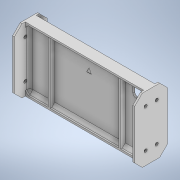
# Autodesk Inventor part: screen cover backplate
Saved by Autodesk Inventor 2021 (Build 250183000, 183)
## iProperties
Created: 2022-01-29
Part Number: screen cover backplate
Material: Generic
Document SubType Name: Modeling
Designer: Toby
Density: 1 g/cm^3
Appearance: Default
Author: Toby
Autodesk Inventor part; units mm, degrees
ref_plane "YZ Plane" through (0, 0, 0) normal (1, 0, 0) x (0, 1, 0)
ref_plane "XZ Plane" through (0, 0, 0) normal (0, 1, 0) x (-1, 0, 0)
ref_plane "XY Plane" through (0, 0, 0) normal (0, 0, 1) x (1, 0, 0)
sketch "Sketch1" plane through (0, 0, 0) normal (0, 0, 1) x (1, 0, 0)
  line L0 (-49.4736, 23.6675) -> (30.5264, 23.6675)
  line L1 (30.5264, 23.6675) -> (30.5264, -18.3325)
  line L2 (30.5264, -18.3325) -> (-49.4736, -18.3325)
  line L3 (-49.4736, -18.3325) -> (-49.4736, 23.6675)
  line L4 (-47.9736, 22.4675) -> (29.0264, 22.4675)
  line L5 (29.0264, 22.4675) -> (29.0264, -17.1325)
  line L6 (29.0264, -17.1325) -> (-47.9736, -17.1325)
  line L7 (-47.9736, -17.1325) -> (-47.9736, 22.4675)
  point P0 (0, 0)
  dimension "d0" = 80
  dimension "d1" = 42
  dimension "d2" = 1.5
  dimension "d3" = 1.5
  dimension "d4" = 1.2
  dimension "d5" = 1.2
  constraints: 16 end point, 4 parallel, 2 horizontal, 2 perpendicular
  measures "d0" distance of L0.start L0.end
  measures "d1" distance of L2.end L0.start
  measures "d2" distance between parallel lines of L7 L3
  measures "d3" distance between parallel lines of L1 L5
  measures "d4" distance between parallel lines of L0 L4
  measures "d5" distance between parallel lines of L2 L6
extrude "Extrusion1" add sketch "Sketch1" along normal blind 10
sketch "Sketch2" plane through (0, 0, 10) normal (0, 0, 1) x (1, 0, 0)
  line L0 (-47.9736, -18.3325) -> (29.0264, -18.3325)
  line L1 (29.0264, -18.3325) -> (29.0264, 23.6675)
  line L2 (29.0264, 23.6675) -> (-47.9736, 23.6675)
  line L3 (-47.9736, 23.6675) -> (-47.9736, -18.3325)
  line L4 (-47.9736, -17.1325) -> (-47.9736, 22.4675) projected
  line L5 (29.0264, 22.4675) -> (29.0264, -17.1325) projected
  line L6 (30.5264, 23.6675) -> (-49.4736, 23.6675) projected
  line L7 (-49.4736, -18.3325) -> (30.5264, -18.3325) projected
  point P0 (0, 0)
  constraints: 8 end point, 4 collinear, 2 parallel, 1 horizontal, 1 perpendicular
extrude "Extrusion2" cut sketch "Sketch2" against normal blind 10
sketch "Sketch3" plane through (0, 0, 10) normal (0, 0, 1) x (1, 0, 0)
  line L0 (-60.7413, 24.2408) -> (-49.3736, 24.2408)
  line L1 (-49.3736, 24.2408) -> (-49.3736, -19.8756)
  line L2 (-49.3736, -19.8756) -> (-60.7413, -19.8756)
  line L3 (-60.7413, -19.8756) -> (-60.7413, 24.2408)
  line L4 (46.8098, -23.8693) -> (30.4264, -23.8693)
  line L5 (30.4264, -23.8693) -> (30.4264, 25.2624)
  line L6 (30.4264, 25.2624) -> (46.8098, 25.2624)
  line L7 (46.8098, 25.2624) -> (46.8098, -23.8693)
  line L8 (-49.4736, 23.6675) -> (-49.4736, -18.3325) projected
  line L9 (30.5264, -18.3325) -> (30.5264, 23.6675) projected
  point P0 (0, 0)
  dimension "d10" = 0.1
  dimension "d11" = 0.1
  constraints: 16 end point, 4 parallel, 2 horizontal, 2 perpendicular
  measures "d10" distance between parallel lines of L1 L8
  measures "d11" distance between parallel lines of L9 L5
extrude "Extrusion3" cut sketch "Sketch3" against normal blind 10
sketch "Sketch4" plane through (30.4264, -18.3325, 10) normal (1, 0, 0) x (0, 0, -1)
  line L0 (10, 42) -> (10, 0) projected
  line L1 (0, 42) -> (10, 42) projected
  line L2 (10, 0) -> (0, 0) projected
  point P0 (10, 18.3325)
  point P1 (7, 33.5)
  point P2 (7, 8.5)
  dimension "d14" = 3
  dimension "d15" = 3
  dimension "d16" = 8.5
  dimension "d17" = 8.5
  measures "d14" distance from line of L0 point (7, 33.5)
  measures "d15" distance from line of L0 point (7, 8.5)
  measures "d16" distance from line of L1 point (7, 33.5)
  measures "d17" distance from line of L2 point (7, 8.5)
hole "Hole1" at (30.4264, 15.1675, 3) at (30.4264, -9.8325, 3) direction (-1, 0, 0) diameter 2 depth 10 tip angle 179
sketch "Sketch5" plane through (-49.3736, -18.3325, 10) normal (-1, 0, 0) x (0, 0, 1)
  circle A0 centre (-7, 33.5) radius 1 projected
  circle A1 centre (-7, 8.5) radius 1 projected
  point P0 (-10, 18.3325)
  constraints: 2 coincident
hole "Hole2" at (-49.3736, 15.1675, 3) at (-49.3736, -9.8325, 3) direction (1, 0, 0) diameter 2 depth 10 tip angle 179
chamfer "Chamfer1" distance 5 angle 45 4 edges at (-48.6736, 23.6675, 10) (-48.6736, -18.3325, 10) (29.7264, -18.3325, 10) (29.7264, 23.6675, 10)
sketch "Sketch6" plane through (0, 0, 0) normal (0, 0, -1) x (-1, 0, 0)
  line L0 (-30.4264, 23.6675) -> (-30.4264, -18.3325) projected
  line L1 (49.3736, -18.3325) -> (47.9736, -18.3325) projected
  line L2 (-30.4264, 23.6675) -> (49.3736, 23.6675)
  line L3 (49.3736, 23.6675) -> (49.3736, -18.3325)
  line L4 (49.3736, -18.3325) -> (-30.4264, -18.3325)
  line L5 (-30.4264, -18.3325) -> (-30.4264, 23.6675)
  point P0 (0, 0)
  point P1 (-30.4264, -18.3325)
  constraints: 8 end point, 2 parallel, 1 horizontal, 1 perpendicular
extrude "Extrusion4" add sketch "Sketch6" along normal blind 1.2
sketch "Sketch7" plane through (0, 0, -1.2) normal (0, 0, -1) x (-1, 0, 0)
  line L0 (-29.0264, -18.3325) -> (-29.0264, 23.6675) projected
  line L1 (-29.0264, 23.6675) -> (-19.0264, 23.6675)
  line L2 (-19.0264, 23.6675) -> (-19.0264, 13.6675)
  line L3 (-19.0264, 13.6675) -> (-29.0264, 13.6675)
  line L4 (-29.0264, 13.6675) -> (-29.0264, 23.6675)
  point P0 (0, 0)
  dimension "d37" = 10
  dimension "d38" = 10
  constraints: 8 end point, 2 parallel, 1 horizontal, 1 perpendicular
  measures "d37" distance of L2.end L3.end
  measures "d38" distance of L1.end L2.end
extrude "Extrusion5" cut sketch "Sketch7" against normal blind 1.2
fillet "Fillet1" radius 2 2 edges at (19.0264, 13.6675, -0.6) (29.0264, 13.6675, -0.6)
sketch "Sketch9" plane through (0, 0, 0) normal (0, 0, 1) x (1, 0, 0)
  line L0 (42.1128, -25.2677) -> (-53.8311, -25.2677)
  line L1 (-53.8311, -25.2677) -> (-53.8311, -18.2325)
  line L2 (-53.8311, -18.2325) -> (42.1128, -18.2325)
  line L3 (42.1128, -18.2325) -> (42.1128, -25.2677)
  line L4 (-54.7833, 25.6339) -> (39.9156, 25.6339)
  line L5 (39.9156, 25.6339) -> (39.9156, 23.5675)
  line L6 (39.9156, 23.5675) -> (-54.7833, 23.5675)
  line L7 (-54.7833, 23.5675) -> (-54.7833, 25.6339)
  line L8 (29.0264, -18.3325) -> (-47.9736, -18.3325) projected
  line L9 (-47.9736, 23.6675) -> (19.0264, 23.6675) projected
  point P0 (0, 0)
  dimension "d56" = 0.1
  dimension "d57" = 0.1
  constraints: 16 end point, 4 parallel, 2 horizontal, 2 perpendicular
  measures "d56" distance between parallel lines of L2 L8
  measures "d57" distance between parallel lines of L9 L6
extrude "Extrusion7" cut sketch "Sketch9" along normal mid plane 50
fillet "Fillet2" radius 2 2 edges at (-47.9736, 2.6675, 0) (29.0264, -1.2825, 0)
sketch "Sketch10" plane through (0, 0, 0) normal (0, 0, 1) x (1, 0, 0)
  line L0 (-47.9736, 23.5675) -> (-47.9736, 15.1675) projected
  line L1 (19.0264, 23.5675) -> (19.0264, 15.6675) projected
  line L2 (-47.9736, 23.5675) -> (19.0264, 23.5675)
  line L3 (19.0264, 23.5675) -> (19.0264, 22.4717)
  line L4 (19.0264, 22.4717) -> (-47.9736, 22.4717)
  line L5 (-47.9736, 22.4717) -> (-47.9736, 23.5675)
  line L6 (29.0264, -18.2325) -> (29.0264, -9.8325) projected
  line L7 (-47.9736, -9.8325) -> (-47.9736, -18.2325) projected
  line L8 (29.0264, -18.2325) -> (-47.9736, -18.2325)
  line L9 (-47.9736, -18.2325) -> (-47.9736, -17.0297)
  line L10 (-47.9736, -17.0297) -> (29.0264, -17.0297)
  line L11 (29.0264, -17.0297) -> (29.0264, -18.2325)
  point P0 (0, 0)
  point P1 (29.0264, -17.0297)
  constraints: 16 end point, 4 parallel, 2 horizontal, 2 perpendicular, 2 point on line
extrude "Extrusion8" add sketch "Sketch10" along normal blind 3
sketch "Sketch13" plane through (0, 0, -1.2) normal (0, 0, -1) x (-1, 0, 0)
  line L0 (-31.9264, 25.0675) -> (50.8736, 25.0675)
  line L1 (50.8736, 25.0675) -> (50.8736, -19.7325)
  line L2 (50.8736, -19.7325) -> (-31.9264, -19.7325)
  line L3 (-31.9264, -19.7325) -> (-31.9264, 25.0675)
  line L4 (49.3736, 23.5675) -> (-19.0264, 23.5675) projected
  line L5 (-30.4264, -18.2325) -> (49.3736, -18.2325) projected
  line L6 (-30.4264, 23.5675) -> (-30.4264, -18.2325) projected
  line L7 (49.3736, -18.2325) -> (49.3736, 23.5675) projected
  line L8 (-30.4264, 23.5675) -> (49.3736, 23.5675)
  line L9 (49.3736, 23.5675) -> (49.3736, -18.2325)
  line L10 (49.3736, -18.2325) -> (-30.4264, -18.2325)
  line L11 (-30.4264, -18.2325) -> (-30.4264, 23.5675)
  point P0 (0, 0)
  dimension "d81" = 1.5
  dimension "d82" = 1.5
  dimension "d83" = 1.5
  dimension "d84" = 1.5
  constraints: 16 end point, 4 parallel, 2 horizontal, 2 perpendicular
  measures "d81" distance between parallel lines of L4 L0
  measures "d82" distance between parallel lines of L2 L5
  measures "d83" distance between parallel lines of L6 L3
  measures "d84" distance between parallel lines of L7 L1
extrude "Extrusion11" add sketch "Sketch13" against normal blind 1.2
fillet "Fillet3" radius 2 3 edges at (31.9264, 25.0675, -0.6) (-50.8736, 25.0675, -0.6) (31.9264, -19.7325, -0.6)
fillet "Fillet4" radius 2 1 edges at (-50.8736, -19.7325, -0.6)
sketch "Sketch14" plane through (0, 0, -1.2) normal (0, 0, -1) x (-1, 0, 0)
  line L0 (-30.4264, 23.5675) -> (-29.0264, 23.5675) projected
  line L1 (-30.4264, -18.2325) -> (-30.4264, 23.5675) projected
  line L2 (-29.0264, 23.5675) -> (-30.4264, 23.5675)
  line L3 (-30.4264, 23.5675) -> (-30.4264, -18.2325)
  line L4 (-30.4264, -18.2325) -> (-29.0264, -18.2325)
  line L5 (-29.0264, -18.2325) -> (-29.0264, 23.5675)
  line L6 (49.3736, -18.2325) -> (47.9736, -18.2325) projected
  line L7 (49.3736, 23.5675) -> (49.3736, -18.2325) projected
  line L8 (47.9736, -18.2325) -> (49.3736, -18.2325)
  line L9 (49.3736, -18.2325) -> (49.3736, 23.5675)
  line L10 (49.3736, 23.5675) -> (47.9736, 23.5675)
  line L11 (47.9736, 23.5675) -> (47.9736, -18.2325)
  line L12 (-31.9264, 23.0675) -> (-31.9264, -17.7325) projected
  line L13 (48.8736, 25.0675) -> (-29.9264, 25.0675) projected
  point P0 (0, 0)
  dimension "d89" = 1.5
  dimension "d90" = 1.5
  constraints: 16 end point, 4 parallel, 2 horizontal, 2 perpendicular
  measures "d89" distance between parallel lines of L12 L1
  measures "d90" distance from line of L13 L0.start
extrude "Extrusion12" add sketch "Sketch14" along normal blind 10
sketch "Sketch15" plane through (30.4264, -18.2325, -1.2) normal (1, 0, 0) x (0, 0, -1)
  line L0 (0, 41.8) -> (10, 41.8) projected
  line L1 (0, 0) -> (10, 0) projected
  line L2 (0, 41.3) -> (0, 0.5) projected
  point P0 (-1.2, 18.2325)
  point P1 (3, 33.3)
  point P2 (3, 8.5)
  point P3 (5, 41.8)
  point P4 (5, 0)
  dimension "d96" = 8.5
  dimension "d97" = 8.5
  dimension "d98" = 3
  dimension "d99" = 3
  measures "d96" distance from line of L0 point (3, 33.3)
  measures "d97" distance from line of L1 point (3, 8.5)
  measures "d98" distance from line of L2 point (3, 8.5)
  measures "d99" distance from line of L2 point (3, 33.3)
hole "Hole3" at (30.4264, 15.0675, -4.2) at (30.4264, -9.7325, -4.2) direction (-1, 0, 0) diameter 2 depth 10 tip angle 179
sketch "Sketch16" plane through (-49.3736, -18.2325, -1.2) normal (-1, 0, 0) x (0, 0, 1)
  circle A0 centre (-3, 33.3) radius 1 projected
  circle A1 centre (-3, 8.5) radius 1 projected
  point P0 (1.2, 18.2325)
  constraints: 2 coincident
hole "Hole4" at (-49.3736, 15.0675, -4.2) at (-49.3736, -9.7325, -4.2) direction (1, 0, 0) diameter 2 depth 10 tip angle 179
chamfer "Chamfer4" distance 5 angle 45 4 edges at (29.7264, 23.5675, -11.2) (-48.6736, 23.5675, -11.2) (29.7264, -18.2325, -11.2) (-48.6736, -18.2325, -11.2)
chamfer "Chamfer5" distance 2 angle 45 5 edges at (-9.4736, -17.0297, 0) (28.4408, -17.0297, 0.5856) (29.0264, -17.0297, 2.4998) (-47.3879, -17.0297, 0.5856) (-47.9736, -17.0297, 2.4998)
chamfer "Chamfer6" distance 2 angle 45 2 edges at (-13.4738, 22.4717, 0) (-47.3879, 22.4717, 0.5856)
sketch "Sketch17" plane through (0, 0, -1.2) normal (0, 0, -1) x (-1, 0, 0)
  line L0 (-19.0264, 23.5675) -> (47.9736, 23.5675) projected
  line L1 (47.9736, 23.5675) -> (-19.0264, 23.5675)
  line L2 (-19.0264, 23.5675) -> (-19.0264, 22.3675)
  line L3 (-19.0264, 22.3675) -> (47.9736, 22.3675)
  line L4 (47.9736, 22.3675) -> (47.9736, 23.5675)
  line L5 (-29.0264, -15.0297) -> (-29.0264, -18.2325) projected
  line L6 (-29.0264, -18.2325) -> (47.9736, -18.2325)
  line L7 (47.9736, -18.2325) -> (47.9736, -17.0325)
  line L8 (47.9736, -17.0325) -> (-29.0264, -17.0325)
  line L9 (-29.0264, -17.0325) -> (-29.0264, -18.2325)
  line L10 (-19.0264, 23.5675) -> (-19.0264, 15.6675) projected
  point P0 (0, 0)
  point P1 (-29.0264, -17.0325)
  dimension "d123" = 1.2
  dimension "d124" = 1.2
  constraints: 16 end point, 4 parallel, 2 horizontal, 2 perpendicular, 1 collinear, 1 point on line
  measures "d123" distance between parallel lines of L3 L0
  measures "d124" distance between parallel lines of L6 L8
extrude "Extrusion13" add sketch "Sketch17" along normal blind 3
chamfer "Chamfer7" distance 2 angle 45 1 edges at (-14.4736, 22.3675, -1.2)
chamfer "Chamfer8" distance 2 angle 45 1 edges at (-9.4736, -17.0325, -1.2)
sketch "Sketch19" plane through (0, 0, -1.2) normal (0, 0, -1) x (-1, 0, 0)
  line L0 (-30.4264, -18.2325) -> (-30.4264, 23.5675) projected
  line L1 (47.9736, -18.2325) -> (49.3736, -18.2325) projected
  line L2 (-30.4264, 23.5675) -> (49.3736, 23.5675)
  line L3 (49.3736, 23.5675) -> (49.3736, -18.2325)
  line L4 (49.3736, -18.2325) -> (-30.4264, -18.2325)
  line L5 (-30.4264, -18.2325) -> (-30.4264, 23.5675)
  line L6 (55.2974, -21.7914) -> (-35.5213, -21.7914)
  line L7 (-35.5213, -21.7914) -> (-35.5213, 27.2078)
  line L8 (-35.5213, 27.2078) -> (55.2974, 27.2078)
  line L9 (55.2974, 27.2078) -> (55.2974, -21.7914)
  point P0 (0, 0)
  constraints: 16 end point, 4 parallel, 2 horizontal, 2 perpendicular
extrude "Extrusion14" cut sketch "Sketch19" against normal blind 3
sketch "Sketch20" plane through (0, 0, -1.2) normal (0, 0, -1) x (-1, 0, 0)
  line L0 (-19.0264, 22.4717) -> (45.9736, 22.4717) projected
  line L1 (-27.0264, -17.0297) -> (45.9736, -17.0297) projected
  line L2 (-14.0264, 22.4717) -> (-12.8264, 22.4717)
  line L3 (-12.8264, 22.4717) -> (-12.8264, -17.0297)
  line L4 (-12.8264, -17.0297) -> (-14.0264, -17.0297)
  line L5 (-14.0264, -17.0297) -> (-14.0264, 22.4717)
  line L6 (31.7736, 22.4717) -> (32.9736, 22.4717)
  line L7 (32.9736, 22.4717) -> (32.9736, -17.0297)
  line L8 (32.9736, -17.0297) -> (31.7736, -17.0297)
  line L9 (31.7736, -17.0297) -> (31.7736, 22.4717)
  line L10 (-29.0264, -13.2325) -> (-29.0264, 18.5675) projected
  line L11 (47.9736, 18.5675) -> (47.9736, -13.2325) projected
  point P0 (0, 0)
  point P1 (32.9736, -17.0297)
  dimension "d135" = 1.2
  dimension "d136" = 1.2
  dimension "d137" = 15
  dimension "d138" = 15
  constraints: 16 end point, 4 parallel, 4 point on line, 2 horizontal, 2 perpendicular
  measures "d135" distance between parallel lines of L3 L5
  measures "d136" distance between parallel lines of L7 L9
  measures "d137" distance between parallel lines of L10 L5
  measures "d138" distance between parallel lines of L11 L7
extrude "Extrusion15" add sketch "Sketch20" along normal blind 3 contours L0 L3 L1 L5 | L0 L7 L1 L9
sketch "Sketch21" plane through (0, 0, 0) normal (0, 0, 1) x (1, 0, 0)
  line L0 (-32.9736, 22.3675) -> (-32.9736, 20.3675) projected
  line L1 (-32.9736, -17.0297) -> (-31.7736, -17.0297) projected
  line L2 (-32.9736, 22.3675) -> (-31.7736, 22.3675)
  line L3 (-31.7736, 22.3675) -> (-31.7736, -17.0297)
  line L4 (-31.7736, -17.0297) -> (-32.9736, -17.0297)
  line L5 (-32.9736, -17.0297) -> (-32.9736, 22.3675)
  line L6 (14.0264, 22.3675) -> (14.0264, -17.0297) projected
  line L7 (12.8264, -17.0297) -> (12.8264, 22.3675) projected
  line L8 (14.0264, -17.0297) -> (12.8264, -17.0297)
  line L9 (12.8264, -17.0297) -> (12.8264, 22.3675)
  line L10 (12.8264, 22.3675) -> (14.0264, 22.3675)
  line L11 (14.0264, 22.3675) -> (14.0264, -17.0297)
  point P0 (0, 0)
  constraints: 16 end point, 4 parallel, 2 horizontal, 2 perpendicular
extrude "Extrusion16" add sketch "Sketch21" along normal blind 3
sketch "Sketch22" plane through (0, 0, -11.2) normal (0, 0, -1) x (-1, 0, 0)
  line L0 (-43.9257, 27.8444) -> (-30.2264, 27.8444)
  line L1 (-30.2264, 27.8444) -> (-30.2264, -19.4315)
  line L2 (-30.2264, -19.4315) -> (-43.9257, -19.4315)
  line L3 (-43.9257, -19.4315) -> (-43.9257, 27.8444)
  line L4 (58.4435, 29.8546) -> (49.1736, 29.8546)
  line L5 (49.1736, 29.8546) -> (49.1736, -19.4315)
  line L6 (49.1736, -19.4315) -> (58.4435, -19.4315)
  line L7 (58.4435, -19.4315) -> (58.4435, 29.8546)
  line L8 (-30.4264, 23.5675) -> (-30.4264, 18.5675) projected
  line L9 (49.3736, 18.5675) -> (49.3736, 23.5675) projected
  point P0 (0, 0)
  dimension "d143" = 0.2
  dimension "d144" = 0.2
  constraints: 16 end point, 4 parallel, 2 horizontal, 2 perpendicular, 1 point on line
  measures "d143" distance between parallel lines of L8 L1
  measures "d144" distance between parallel lines of L9 L5
extrude "Extrusion17" cut sketch "Sketch22" against normal blind 30
sketch "Sketch23" plane through (-47.9736, 23.5675, 3) normal (0, 1, 0) x (1, 0, 0)
  line L0 (67, 7.2) -> (67, 0) projected
  line L1 (0, 7.2) -> (77, 7.2) projected
  line L2 (67, 0) -> (77, 0)
  line L3 (77, 0) -> (77, 7.2)
  line L4 (77, 7.2) -> (67, 7.2)
  line L5 (67, 7.2) -> (67, 0)
  point P0 (47.9736, 3)
  constraints: 8 end point, 2 parallel, 1 horizontal, 1 perpendicular
extrude "Extrusion18" add sketch "Sketch23" against normal blind 1.2
sketch "Sketch24" plane through (0, 0, 0) normal (0, 0, 1) x (1, 0, 0)
  line L0 (-31.7736, 20.4717) -> (12.8264, 20.4717) projected
  line L1 (-9.4736, 15.4717) -> (-7.9736, 12.4717)
  line L2 (-7.9736, 12.4717) -> (-11.0743, 12.4717)
  line L3 (-11.0743, 12.4717) -> (-9.4736, 15.4717)
  point P0 (0, 0)
  point P1 (-9.4736, 20.4717)
  dimension "d149" = 3
  dimension "d150" = 3
  dimension "d151" = 1.5
  dimension "d152" = 0
  dimension "d153" = 5
  constraints: 6 end point, 1 horizontal, 1 midpoint
  measures "d149" vertical distance of L1.start L1.end
  measures "d150" vertical distance of L1.start L2.end
  measures "d151" horizontal distance of L1.start L1.end
  measures "d152" horizontal distance of point (-9.474, 20.472) L1.start
  measures "d153" distance of point (-9.474, 20.472) L1.start
extrude "Extrusion19" cut sketch "Sketch24" against normal blind 0.2
body "Solid1"
